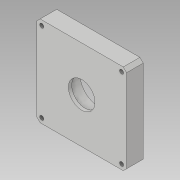
# Autodesk Inventor part: bearing_mount_part_2
Saved by Autodesk Inventor 2017 (Build 210142000, 142)
## iProperties
Part Number: bearing_mount_part_2
Material: Generisch
Document SubType Name: Modeling
Designer: Max
Density: 1 g/cm^3
Appearance: Vorgabe
Mass: 24.0743 g
Surface Area: 85.1839 cm^2
Volume: 24.0743 cm^3
Author: Max
Autodesk Inventor part; units mm, degrees
ref_plane "YZ Plane" through (0, 0, 0) normal (1, 0, 0) x (0, 1, 0)
ref_plane "XZ Plane" through (0, 0, 0) normal (0, 1, 0) x (-1, 0, 0)
ref_plane "XY Plane" through (0, 0, 0) normal (0, 0, 1) x (1, 0, 0)
sketch "Skizze1" plane through (0, 0, 0) normal (0, 1, 0) x (-1, 0, 0)
  line L0 (-27, 27) -> (27, 27)
  line L1 (27, 27) -> (27, -27)
  line L2 (27, -27) -> (-27, -27)
  line L3 (-27, -27) -> (-27, 27)
  line L4 (-27, 27) -> (27, -27) construction
  line L5 (27, 27) -> (-27, -27) construction
  point P0 (0, 0)
  dimension "d0" = 54
  dimension "d1" = 54
  constraints: 12 end point, 2 midpoint, 2 parallel, 1 horizontal, 1 perpendicular
  measures "d0" distance of L1.end L2.end
  measures "d1" distance of L0.end L1.end
extrude "Extrusion1" add sketch "Skizze1" along normal blind 10
chamfer "Fase1" distance 2 angle 45 4 edges at (27, 5, 27) (27, 5, -27) (-27, 5, 27) (-27, 5, -27)
sketch "Skizze2" plane through (0, 10, 0) normal (0, 1, 0) x (1, 0, 0)
  circle A0 centre (0, 0) radius 11
  dimension "d7" = 22
  constraints: 1 centre point, 1 coincident
  measures "d7" diameter of A0
extrude "Extrusion2" cut sketch "Skizze2" against normal blind 8
sketch "Skizze5" plane through (0, 0, 0) normal (0, -1, 0) x (1, 0, 0)
  line L0 (-24, -24) -> (24, -24)
  line L1 (24, -24) -> (24, 24)
  line L2 (24, 24) -> (-24, 24)
  line L3 (-24, 24) -> (-24, -24)
  line L4 (-24, -24) -> (24, 24) construction
  line L5 (24, -24) -> (-24, 24) construction
  point P0 (0, 0)
  dimension "d22" = 48
  dimension "d23" = 48
  constraints: 12 end point, 2 midpoint, 2 parallel, 1 horizontal, 1 perpendicular
  measures "d22" distance of L1.end L2.end
  measures "d23" distance of L0.end L1.end
hole "Bohrung2" at (-24, 0, -24) at (-24, 0, 24) at (24, 0, 24) at (24, 0, -24) direction (0, 1, 0) diameter 2.459 end through all thread size "M3x0.5" class "6H" standard "ISO Metric profile"
sketch "Skizze6" plane through (0, 0, 0) normal (0, -1, 0) x (1, 0, 0)
  circle A0 centre (0, 0) radius 8
  dimension "d31" = 16
  constraints: 1 centre point, 1 coincident
  measures "d31" diameter of A0
extrude "Extrusion4" cut sketch "Skizze6" against normal through all
sketch "Skizze7" plane through (0, 10, 0) normal (0, 1, 0) x (1, 0, 0)
  circle A0 centre (24, -24) radius 1.2295 projected
  circle A1 centre (-24, 24) radius 1.2295 projected
  circle A2 centre (-24, -24) radius 1.2295 projected
  circle A3 centre (24, 24) radius 1.2295 projected
  circle A4 centre (0, 0) radius 11 projected
  line L0 (-27, 25) -> (-25, 27) projected
  line L1 (-27, 25) -> (-27, -25) projected
  line L2 (-25, -27) -> (-27, -25) projected
  line L3 (-25, -27) -> (25, -27) projected
  line L4 (27, -25) -> (25, -27) projected
  line L5 (27, -25) -> (27, 25) projected
  line L6 (25, 27) -> (27, 25) projected
  line L7 (25, 27) -> (-25, 27) projected
  line L8 (-27, -15) -> (-17, -15)
  line L9 (-17, -15) -> (-17, 15)
  line L10 (-17, 15) -> (-27, 15)
  line L11 (-27, 15) -> (-27, -15)
  dimension "d36" = 30
  dimension "d37" = 15
  dimension "d38" = 10
  constraints: 8 end point, 2 parallel, 1 horizontal, 1 perpendicular, 1 point on line
  measures "d36" distance of L8.end L9.end
  measures "d37" distance from line of L8 point (0, 0)
  measures "d38" distance of L8.start L8.end
extrude "Extrusion5" cut sketch "Skizze7" against normal blind 3 contours L10 L9 L8 L1
fillet "Rundung1" radius 2 2 edges at (-17, 8.5, 15) (-17, 8.5, -15)
equation "\"d37\" = 0.5 * d36"
